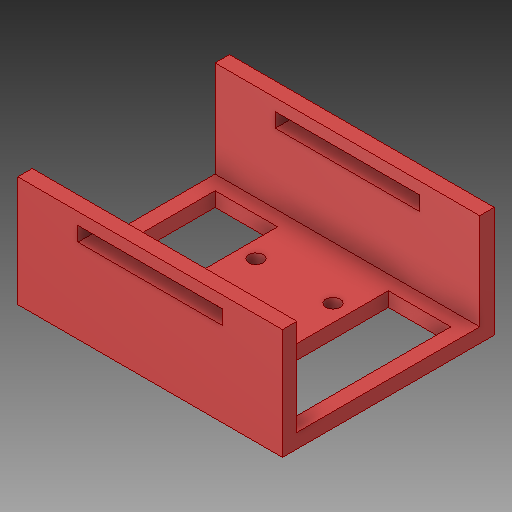
# Autodesk Inventor part: Li-Pol_uchwyt
Saved by Autodesk Inventor 2018 (Build 220112000, 112)
## iProperties
Created: 2018-08-13
Part Number: Li-Pol_uchwyt
Material: Tworzywo sztuczne PET
Document SubType Name: Modeling
Designer: Wojciech
Density: 1.541 g/cm^3
Appearance: Gładki - czerwony
Mass: 16.5491 g
Surface Area: 90.4255 cm^2
Volume: 10.7392 cm^3
Author: Wojciech
Autodesk Inventor part; units mm, degrees
ref_plane "YZ Plane" through (0, 0, 0) normal (1, 0, 0) x (0, 1, 0)
ref_plane "XZ Plane" through (0, 0, 0) normal (0, 1, 0) x (-1, 0, 0)
ref_plane "XY Plane" through (0, 0, 0) normal (0, 0, 1) x (1, 0, 0)
sketch "Szkic1" plane through (0, 0, 0) normal (0, 1, 0) x (-1, 0, 0)
  line L0 (27.5, 22) -> (-27.5, 22)
  line L1 (-27.5, 22) -> (-27.5, -22)
  line L2 (-27.5, -22) -> (27.5, -22)
  line L3 (27.5, -22) -> (27.5, 22)
  line L4 (27.5, 22) -> (-27.5, -22) construction
  line L5 (-27.5, 22) -> (27.5, -22) construction
  point P0 (0, 0)
  dimension "d0" = 55
  dimension "d1" = 44
  constraints: 12 end point, 2 midpoint, 2 parallel, 1 horizontal, 1 perpendicular
  measures "d0" distance of L2.end L1.end
  measures "d1" distance of L1.end L0.end
extrude "Wyciągnięcie proste1" add sketch "Szkic1" along normal blind 3
sketch "Szkic2" plane through (0, 3, 0) normal (0, 1, 0) x (1, 0, 0)
  line L0 (27.5, 22) -> (-27.5, 22) projected
  line L1 (27.5, -22) -> (27.5, 22) projected
  line L2 (-27.5, 22) -> (27.5, 22)
  line L3 (27.5, 22) -> (27.5, 19)
  line L4 (27.5, 19) -> (-27.5, 19)
  line L5 (-27.5, 19) -> (-27.5, 22)
  line L6 (-27.5, 22) -> (-27.5, -22) projected
  line L7 (27.5, -22) -> (-27.5, -22)
  line L8 (-27.5, -22) -> (-27.5, -19)
  line L9 (-27.5, -19) -> (27.5, -19)
  line L10 (27.5, -19) -> (27.5, -22)
  point P0 (0, 0)
  dimension "d4" = 3
  dimension "d5" = 3
  constraints: 16 end point, 4 parallel, 2 horizontal, 2 perpendicular, 2 point on line
  measures "d4" distance of L2.end L3.end
  measures "d5" distance of L7.end L8.end
extrude "Wyciągnięcie proste2" add sketch "Szkic2" along normal blind 20 contours L1 L4 L5 L0 | L1 L7 L6 L9
sketch "Szkic4" plane through (0, 3, 0) normal (0, 1, 0) x (1, 0, 0)
  line L0 (-27.5, 19) -> (-27.5, -19) projected
  line L1 (-27.5, 0) -> (27.5, 0) construction
  line L2 (27.5, -19) -> (27.5, 19) projected
  line L3 (-27.5, -22) -> (27.5, -22) projected
  line L4 (0, -22) -> (0, 22) construction
  line L5 (27.5, 22) -> (-27.5, 22) projected
  point P0 (0, 0)
  point P1 (-8, -8)
  point P2 (-8, 8)
  point P3 (8, -8)
  point P4 (8, 8)
  dimension "d13" = 8
  dimension "d16" = 8
  constraints: 4 end point, 4 midpoint, 3 symmetric about line
  measures "d13" horizontal distance of point (0, 0) point (-8, -8)
  measures "d16" horizontal distance of point (0, 0) point (-8, -8)
hole "Otwór1" at (-8, 3, 8) at (-8, 3, -8) at (8, 3, 8) at (8, 3, -8) direction (0, -1, 0) diameter 3 depth 8 tip angle 118
sketch "Szkic5" plane through (0, 3, 0) normal (0, 1, 0) x (1, 0, 0)
  line L0 (-24.5, -16) -> (-11.5, -16)
  line L1 (-11.5, -16) -> (-11.5, 16)
  line L2 (-11.5, 16) -> (-24.5, 16)
  line L3 (-24.5, 16) -> (-24.5, -16)
  line L4 (27.5, -19) -> (-27.5, -19) projected
  line L5 (27.5, 19) -> (-27.5, 19) projected
  line L6 (-27.5, 22) -> (-27.5, -22) projected
  line L7 (-27.5, -22) -> (27.5, -22) projected
  line L8 (0, -22) -> (0, 22) construction
  line L9 (27.5, 22) -> (-27.5, 22) projected
  line L10 (24.5, -16) -> (11.5, -16)
  line L11 (11.5, -16) -> (11.5, 16)
  line L12 (11.5, 16) -> (24.5, 16)
  line L13 (24.5, 16) -> (24.5, -16)
  point P0 (0, 0)
  dimension "d27" = 3
  dimension "d28" = 3
  dimension "d29" = 3
  dimension "d30" = 13
  constraints: 18 end point, 4 symmetric about line, 2 midpoint, 2 parallel, 1 horizontal, 1 perpendicular
  measures "d27" distance between parallel lines of L4 L0
  measures "d28" distance between parallel lines of L5 L2
  measures "d29" distance between parallel lines of L6 L3
  measures "d30" distance of L1.end L2.end
sketch "Szkic6" plane through (-27.5, 0, 22) normal (0, 0, 1) x (1, 0, 0)
  line L0 (12.5, 17.5) -> (42.5, 17.5)
  line L1 (42.5, 17.5) -> (42.5, 20.5)
  line L2 (42.5, 20.5) -> (12.5, 20.5)
  line L3 (12.5, 20.5) -> (12.5, 17.5)
  line L4 (12.5, 17.5) -> (42.5, 20.5) construction
  line L5 (42.5, 17.5) -> (12.5, 20.5) construction
  line L6 (55, 23) -> (0, 23) projected
  line L7 (55, 0) -> (55, 23) projected
  point P0 (27.5, 0)
  point P1 (27.5, 19)
  dimension "d33" = 30
  dimension "d34" = 3
  dimension "d35" = 4
  dimension "d36" = 27.5
  constraints: 12 end point, 2 midpoint, 2 parallel, 1 horizontal, 1 perpendicular
  measures "d33" distance of L2.end L1.end
  measures "d34" distance of L1.end L0.end
  measures "d35" distance from line of L6 point (27.5, 19)
  measures "d36" distance from line of L7 point (27.5, 19)
extrude "Wyciągnięcie proste4" cut sketch "Szkic6" against normal through all
extrude "Wyciągnięcie proste5" cut sketch "Szkic5" against normal blind 10
